Autodesk Inventor part; units mm, degrees
(part 3 of 3)
sketch "Skizze42" plane through (0, 0, 0) normal (0, 0, -1) x (-1, 0, 0)
  line L0 (-79.15, 73.1454) -> (-79.15, 69.8546)
  line L1 (-82, 74.7909) -> (-79.15, 73.1454)
  line L2 (-79.15, 69.8546) -> (-82, 68.2091)
  line L3 (-82, 68.2091) -> (-84.85, 69.8546)
  line L4 (-84.85, 69.8546) -> (-84.85, 73.1454)
  line L5 (-84.85, 73.1454) -> (-82, 74.7909)
  line L6 (-82, 74.7909) -> (-96.75, 74.7909)
  line L7 (-82, 68.2091) -> (-96.75, 68.2091)
  line L8 (-96.75, 74.7909) -> (-96.75, 68.2091)
  line L9 (-94, 91.5) -> (-70, 91.5) construction
  line L10 (-82, 91.5) -> (-82, -91.5) construction
  line L11 (-70, -91.5) -> (-94, -91.5) construction
  line L12 (-94, -91.5) -> (-94, 91.5) construction
  line L13 (-70, -62) -> (-70, 91.5) construction
  line L14 (-82, 34.7909) -> (-79.15, 33.1454)
  line L15 (-79.15, 33.1454) -> (-79.15, 29.8546)
  line L16 (-79.15, 29.8546) -> (-82, 28.2091)
  line L17 (-82, 28.2091) -> (-84.85, 29.8546)
  line L18 (-84.85, 33.1454) -> (-82, 34.7909)
  line L19 (-84.85, 29.8546) -> (-84.85, 33.1454)
  line L20 (-82, 28.2091) -> (-96.75, 28.2091)
  line L21 (-82, 34.7909) -> (-96.75, 34.7909)
  line L22 (-96.75, 34.7909) -> (-96.75, 28.2091)
  line L23 (-82, -14.7909) -> (-84.85, -13.1454)
  line L24 (-82, -8.2091) -> (-96.75, -8.2091)
  line L25 (-82, -8.2091) -> (-79.15, -9.8546)
  line L26 (-84.85, -9.8546) -> (-82, -8.2091)
  line L27 (-96.75, -8.2091) -> (-96.75, -14.7909)
  line L28 (-82, -14.7909) -> (-96.75, -14.7909)
  line L29 (-84.85, -13.1454) -> (-84.85, -9.8546)
  line L30 (-79.15, -9.8546) -> (-79.15, -13.1454)
  line L31 (-79.15, -13.1454) -> (-82, -14.7909)
  line L32 (-82, -54.7909) -> (-84.85, -53.1454)
  line L33 (-82, -48.2091) -> (-96.75, -48.2091)
  line L34 (-82, -48.2091) -> (-79.15, -49.8546)
  line L35 (-84.85, -49.8546) -> (-82, -48.2091)
  line L36 (-96.75, -48.2091) -> (-96.75, -54.7909)
  line L37 (-82, -54.7909) -> (-96.75, -54.7909)
  line L38 (-84.85, -53.1454) -> (-84.85, -49.8546)
  line L39 (-79.15, -49.8546) -> (-79.15, -53.1454)
  line L40 (-79.15, -53.1454) -> (-82, -54.7909)
  line L41 (0, 91.5) -> (0, -95.2854)
  line L42 (79.15, 73.1454) -> (79.15, 69.8546)
  line L43 (82, 74.7909) -> (79.15, 73.1454)
  line L44 (79.15, 69.8546) -> (82, 68.2091)
  line L45 (82, 68.2091) -> (84.85, 69.8546)
  line L46 (84.85, 69.8546) -> (84.85, 73.1454)
  line L47 (84.85, 73.1454) -> (82, 74.7909)
  line L48 (82, 74.7909) -> (96.75, 74.7909)
  line L49 (96.75, 74.7909) -> (96.75, 68.2091)
  line L50 (94, 91.5) -> (70, 91.5) construction
  line L51 (82, 68.2091) -> (96.75, 68.2091)
  line L52 (82, 34.7909) -> (96.75, 34.7909)
  line L53 (82, 34.7909) -> (79.15, 33.1454)
  line L54 (84.85, 33.1454) -> (82, 34.7909)
  line L55 (96.75, 34.7909) -> (96.75, 28.2091)
  line L56 (82, 28.2091) -> (96.75, 28.2091)
  line L57 (79.15, 33.1454) -> (79.15, 29.8546)
  line L58 (79.15, 29.8546) -> (82, 28.2091)
  line L59 (82, 28.2091) -> (84.85, 29.8546)
  line L60 (70, -62) -> (70, 91.5) construction
  line L61 (82, 91.5) -> (82, -91.5) construction
  line L62 (94, -91.5) -> (94, 91.5) construction
  line L63 (70, -91.5) -> (94, -91.5) construction
  line L64 (84.85, 29.8546) -> (84.85, 33.1454)
  line L65 (82, -8.2091) -> (79.15, -9.8546)
  line L66 (84.85, -9.8546) -> (82, -8.2091)
  line L67 (79.15, -9.8546) -> (79.15, -13.1454)
  line L68 (84.85, -13.1454) -> (84.85, -9.8546)
  line L69 (82, -14.7909) -> (84.85, -13.1454)
  line L70 (79.15, -13.1454) -> (82, -14.7909)
  line L71 (82, -48.2091) -> (79.15, -49.8546)
  line L72 (79.15, -49.8546) -> (79.15, -53.1454)
  line L73 (79.15, -53.1454) -> (82, -54.7909)
  line L74 (82, -8.2091) -> (96.75, -8.2091)
  line L75 (82, -54.7909) -> (84.85, -53.1454)
  line L76 (84.85, -49.8546) -> (82, -48.2091)
  line L77 (84.85, -53.1454) -> (84.85, -49.8546)
  line L78 (96.75, -8.2091) -> (96.75, -14.7909)
  line L79 (82, -14.7909) -> (96.75, -14.7909)
  line L80 (82, -48.2091) -> (96.75, -48.2091)
  line L81 (96.75, -48.2091) -> (96.75, -54.7909)
  line L82 (82, -54.7909) -> (96.75, -54.7909)
  circle A0 centre (82, 71.5) radius 1.7
  circle A1 centre (82, 31.5) radius 1.7
  circle A2 centre (82, -11.5) radius 1.7
  circle A3 centre (82, -51.5) radius 1.7
  circle A4 centre (-82, -51.5) radius 1.7
  circle A5 centre (-82, -11.5) radius 1.7
  circle A6 centre (-82, 31.5) radius 1.7
  circle A7 centre (-82, 71.5) radius 1.7
  point P0 (0, 0)
  point P1 (0, 0)
  point P2 (-82, 71.5)
  point P3 (-82, 71.5)
  point P4 (-82, -51.5)
  point P5 (-82, 31.5)
  point P6 (-82, -11.5)
  point P7 (-82, 31.5)
  point P8 (-82, -11.5)
  point P9 (-82, -11.5)
  point P10 (-82, -11.5)
  point P11 (82, 71.5)
  point P12 (82, 31.5)
  point P13 (82, -11.5)
  point P14 (82, -51.5)
  point P15 (82, -51.5)
  point P16 (82, -51.5)
  point P17 (82, -11.5)
  point P18 (82, -11.5)
  point P19 (82, -11.5)
  point P20 (82, -51.5)
  point P21 (82, 31.5)
  point P22 (82, -11.5)
  point P23 (82, -51.5)
  point P24 (-82, -51.5)
  point P25 (-82, -11.5)
  point P26 (-82, 31.5)
  point P27 (-82, 71.5)
  point P28 (-82, 71.5)
  point P29 (-82, 71.5)
  dimension "d202" = 5.7
  dimension "d203" = 12
  dimension "d204" = 12
  dimension "d205" = 20
  dimension "d206" = 40
  dimension "d207" = 40
  dimension "d208" = 40
  dimension "d209" = 5.7
  dimension "d210" = 5.7
  dimension "d211" = 5.7
  dimension "d212" = 3.4
  dimension "d213" = 3.4
  dimension "d214" = 3.4
  dimension "d215" = 3.4
  dimension "d216" = 3.4
  dimension "d217" = 3.4
  dimension "d218" = 3.4
  dimension "d219" = 3.4
  dimension "d220" = 0
  dimension "d221" = 0
  constraints: 166 end point, 8 centre point, 8 point on line, 3 midpoint, 2 coincident, 1 parallel, 1 vertical, 52 other
  measures "d202" distance between parallel lines of L0 L4
  measures "d203" distance between parallel lines of L12 L10
  measures "d204" distance between parallel lines of L10 L13
  measures "d205" distance from line of L9 point (-82, 71.5)
  measures "d206" distance of L10.end point (-82, -51.5)
  measures "d207" distance of point (-82, 31.5) point (-82, 71.5)
  measures "d208" distance of point (-82, -51.5) point (-82, -11.5)
  measures "d209" distance between parallel lines of L15 L19
  measures "d210" distance between parallel lines of L30 L29
  measures "d211" distance between parallel lines of L39 L38
  measures "d212" diameter of A0
  measures "d213" diameter of A1
  measures "d214" diameter of A2
  measures "d215" diameter of A3
  measures "d216" diameter of A4
  measures "d217" diameter of A5
  measures "d218" diameter of A6
  measures "d219" diameter of A7
  measures "d220" distance of point (-82, 71.5) point (-82, 71.5)
  measures "d221" distance of point (82, 71.5) point (82, 71.5)
extrude "Extrusion26" cut sketch "Skizze42" against normal through all contours A0 | A1 | A2 | A3 | A4 | A5 | A6 | A7
sketch "Skizze43" plane through (0, 0, 0) normal (0, 0, -1) x (-1, 0, 0)
  circle A0 centre (-82, 71.5) radius 1.7 projected
  circle A1 centre (-82, 71.5) radius 3
  circle A2 centre (-82, 31.5) radius 1.7 projected
  circle A3 centre (-82, 31.5) radius 3
  circle A4 centre (-82, -11.5) radius 1.7 projected
  circle A5 centre (-82, -11.5) radius 3
  circle A6 centre (-82, -51.5) radius 1.7 projected
  circle A7 centre (-82, -51.5) radius 3
  circle A8 centre (82, -51.5) radius 1.7 projected
  circle A9 centre (82, -51.5) radius 3
  circle A10 centre (82, -11.5) radius 1.7 projected
  circle A11 centre (82, -11.5) radius 3
  circle A12 centre (82, 31.5) radius 1.7 projected
  circle A13 centre (82, 31.5) radius 3
  circle A14 centre (82, 71.5) radius 1.7 projected
  circle A15 centre (82, 71.5) radius 3
  point P0 (0, 0)
  dimension "d224" = 6
  dimension "d225" = 6
  dimension "d226" = 6
  dimension "d227" = 6
  dimension "d228" = 6
  dimension "d229" = 6
  dimension "d230" = 6
  dimension "d231" = 6
  constraints: 8 centre point, 8 coincident
  measures "d224" diameter of A15
  measures "d225" diameter of A13
  measures "d226" diameter of A11
  measures "d227" diameter of A9
  measures "d228" diameter of A1
  measures "d229" diameter of A3
  measures "d230" diameter of A5
  measures "d231" diameter of A7
extrude "Extrusion27" cut sketch "Skizze43" against normal blind 10 contours A1 | A2 | A3 | A4 | A5 | A6 | A7 | A8 | A9 | A10 | A11 | A12 | A13 | A15
sketch "Skizze45" plane through (-89, -91.5, 0) normal (-1, 0, 0) x (0, 0, 1)
  line L0 (6, 140.25) -> (27, 140.25)
  circle A0 centre (7.5, 68.15) radius 1.5
  circle A1 centre (7.5, 91.05) radius 1.5
  circle A2 centre (7.5, 113.95) radius 1.5
  circle A3 centre (7.5, 136.85) radius 1.5
  point P0 (0, 91.5)
  point P1 (7.5, 140.25)
  point P2 (7.5, 139.85)
  point P3 (7.5, 136.85)
  dimension "d282" = 3
  dimension "d283" = 3
  dimension "d284" = 3
  dimension "d285" = 3
  dimension "d288" = 0
  constraints: 4 centre point, 2 end point
  measures "d282" diameter of A0
  measures "d283" diameter of A1
  measures "d284" diameter of A2
  measures "d285" diameter of A3
  measures "d288" distance of point (7.5, 136.85) A3.centre
extrude "Extrusion28" cut sketch "Skizze45" against normal through all
sketch "Skizze46" plane through (89, -91.5, 24) normal (1, 0, 0) x (0, 0, -1)
  circle A0 centre (16.5, 136.85) radius 1.5 projected
  circle A1 centre (16.5, 136.85) radius 3
  circle A2 centre (16.5, 113.95) radius 1.5 projected
  circle A3 centre (16.5, 113.95) radius 3
  circle A4 centre (16.5, 91.05) radius 1.5 projected
  circle A5 centre (16.5, 91.05) radius 3
  circle A6 centre (16.5, 68.15) radius 1.5 projected
  circle A7 centre (16.5, 68.15) radius 3
  point P0 (24, 91.5)
  dimension "d289" = 6
  dimension "d290" = 6
  dimension "d291" = 6
  dimension "d292" = 6
  constraints: 4 centre point, 4 coincident
  measures "d289" diameter of A1
  measures "d290" diameter of A3
  measures "d291" diameter of A5
  measures "d292" diameter of A7
extrude "Extrusion29" cut sketch "Skizze46" against normal blind 5 contours A0 | A1 | A3 | A5 | A7
sketch "Skizze47" plane through (-89, -91.5, 0) normal (-1, 0, 0) x (0, 0, 1)
  circle A0 centre (7.5, 136.85) radius 3 projected
  circle A1 centre (7.5, 136.85) radius 3
  circle A2 centre (7.5, 113.95) radius 1.5 projected
  circle A3 centre (7.5, 113.95) radius 3
  circle A4 centre (7.5, 91.05) radius 3 projected
  circle A5 centre (7.5, 91.05) radius 3
  circle A6 centre (7.5, 68.15) radius 1.5 projected
  circle A7 centre (7.5, 68.15) radius 3
  point P0 (0, 91.5)
  constraints: 4 centre point, 4 coincident
extrude "Extrusion30" cut sketch "Skizze47" against normal blind 5 contours A0 | A2 | A3 | A4 | A6 | A7
